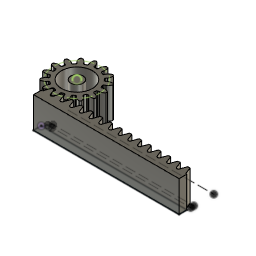
Rack and Gear (For creating a rack and gear) (Autodesk Fusion 360 design; units mm, degrees)
description: Spur Gear; Module: 2.0; Num Teeth: 15; Pressure Angle: 20.0; Backlash: 0.15 mm
Autodesk Fusion 360 part; units mm, degrees
sketch "Sketch1" plane through (0, 0, 0) normal (0, 0, 1) x (1, 0, 0)
  line L0 (0, 0) -> (94.2478, 0)
  line L1 (94.2478, 0) -> (94.2478, -5)
  line L2 (94.2478, -5) -> (0, -5)
  line L3 (0, -5) -> (0, 0)
  line L4 (0, 2.5) -> (94.2478, 2.5) construction
  line L5 (0, 4.5) -> (94.2478, 4.5) construction
  line L6 (0.7359, 0) -> (2.3737, 4.5)
  line L7 (2.3737, 4.5) -> (3.9094, 4.5)
  line L8 (3.9094, 4.5) -> (5.5473, 0)
  line L9 (0, 17.5) -> (94.2478, 17.5) construction
  point P0 (4.6374, 2.5)
  point P1 (1.6458, 2.5)
  point P2 (3.1416, 4.5)
  dimension "d7" = 94.2478
  dimension "d8" = 5
  dimension "d9" = 2.5
  dimension "d10" = 2
  dimension "d11" = 70
  dimension "d12" = 70
  dimension "d13" = 2.9916
  dimension "d14" = 3.1416
  dimension "d43" = 15
  constraint horizontal L0
  constraint vertical L1
  constraint horizontal L2
  constraint vertical L3
  constraint coincident L0.start L3.end
  constraint perpendicular L3 L4
  constraint horizontal L5
  constraint coincident L3 L4.start
  constraint coincident L3 L5.start
  constraint equal L0 L4
  constraint equal L0 L5
  constraint coincident L0 L6.start
  constraint coincident L5 L6.end
  constraint coincident L5 L7.end
  constraint coincident L0 L8.end
  constraint coincident L8 P0
  constraint coincident L4 P0
  constraint coincident L4 P1
  constraint coincident L6 P1
  constraint midpoint L7 P2
  constraint horizontal L9
  constraint equal L0 L9
  constraint coincident L3 L9.start
  measures "d7" distance of L0.start L0.end
  measures "d8" distance of L0.start L2.end
  measures "d9" distance of L0 L4
  measures "d10" distance of L4 L5
  measures "d11" angle of L0 L6
  measures "d12" angle of L0 L8
  measures "d13" distance of P0 P1
  measures "d14" distance of L3 P2
  measures "d43" distance of L4 L9
extrude "Extrude1" add sketch "Sketch1" along normal blind 20 contours L0 L1 L2 L3 makes body 1
extrude "Extrude2" add sketch "Sketch1" along normal blind 20 contours L0 L6 L7 L8 bodies 1
fillet "Fillet1" radius 0.76 2 edges at (0.7359, 0, 10) (5.5473, 0, 10) on bodies 1
pattern_linear "R-Pattern1" count 15 spacing 6.2832 along (1, 0, 0) of "Extrude2", "Fillet1"
copy_body "Body->Comp1" bodies 1 removing the originals makes body 2 in component "rack"
sketch "Sketch1 (2)" plane through (0, 0, 0) normal (0, 0, 1) x (1, 0, 0) in component "Shaft"
  circle A0 centre (0, 0) radius 4
  dimension "d34" = 8
  constraint coincident A0.centre origin
  measures "d34" diameter of A0
extrude "Extrude1'" add sketch "Sketch1 (2)" along normal blind 20 separate body makes body 3 in component "Shaft"
sketch "Sketch1 (3)" plane through (0, 0, 0) normal (0, 0, 1) x (1, 0, 0) in component "Spur Gear (15 teeth)"
  circle A0 centre (0, 0) radius 12.5492
  circle A1 centre (0, 0) radius 10
extrude "Extrude1''" add sketch "Sketch1 (3)" along normal blind 20 separate body makes body 4 in component "Spur Gear (15 teeth)"
sketch "Sketch2" plane through (0, 0, 0) normal (0, 0, 1) x (1, 0, 0) in component "Spur Gear (15 teeth)"
  spline S0 degree 5 poles (13.9988, -1.6471) (14.0073, -1.6481) (14.0244, -1.6499) (14.05, -1.6517) (14.0843, -1.6528) (14.1272, -1.6522) (14.1702, -1.6502) (14.2133, -1.6473) (14.2564, -1.644) (14.2995, -1.6403) (14.3427, -1.6363) (14.3859, -1.6318) (14.4291, -1.6268) (14.4723, -1.621) (14.5156, -1.6146) (14.5589, -1.6075) (14.6022, -1.5999) (14.6454, -1.5918) (14.6887, -1.5833) (14.732, -1.5744) (14.7753, -1.5652) (14.8186, -1.5555) (14.8619, -1.5454) (14.9052, -1.5349) (14.9484, -1.524) (14.9917, -1.5126) (15.0349, -1.5009) (15.0782, -1.4887) (15.1214, -1.4762) (15.1646, -1.4634) (15.2077, -1.4502) (15.2509, -1.4366) (15.294, -1.4227) (15.3372, -1.4084) (15.3803, -1.3938) (15.4233, -1.3789) (15.4664, -1.3636) (15.5094, -1.348) (15.5524, -1.332) (15.5953, -1.3157) (15.6383, -1.2991) (15.6811, -1.2822) (15.724, -1.265) (15.7668, -1.2475) (15.8096, -1.2296) (15.8524, -1.2115) (15.8951, -1.193) (15.9378, -1.1743) (15.9804, -1.1552) (16.023, -1.1359) (16.0655, -1.1162) (16.108, -1.0963) (16.1505, -1.0761) (16.1929, -1.0556) (16.2353, -1.0348) (16.2776, -1.0137) (16.3199, -0.9924) (16.3621, -0.9707) (16.4043, -0.9488) (16.4464, -0.9266) (16.4885, -0.9042) (16.5305, -0.8814) (16.5725, -0.8584) (16.6144, -0.8351) (16.6562, -0.8116) (16.698, -0.7878) (16.7398, -0.7637) (16.7814, -0.7394) (16.8231, -0.7148) (16.8646, -0.6899) (16.9061, -0.6648) (16.9393, -0.6445) (16.9641, -0.6292) (16.9806, -0.6189) (16.9889, -0.6138) knots 0 0 0 0 0 0 0.01428571 0.02857143 0.04285714 0.05714286 0.07142857 0.08571429 0.1 0.11428571 0.12857143 0.14285714 0.15714286 0.17142857 0.18571429 0.2 0.21428571 0.22857143 0.24285714 0.25714286 0.27142857 0.28571429 0.3 0.31428571 0.32857143 0.34285714 0.35714286 0.37142857 0.38571429 0.4 0.41428571 0.42857143 0.44285714 0.45714286 0.47142857 0.48571429 0.5 0.51428571 0.52857143 0.54285714 0.55714286 0.57142857 0.58571429 0.6 0.61428571 0.62857143 0.64285714 0.65714286 0.67142857 0.68571429 0.7 0.71428571 0.72857143 0.74285714 0.75714286 0.77142857 0.78571429 0.8 0.81428571 0.82857143 0.84285714 0.85714286 0.87142857 0.88571429 0.9 0.91428571 0.92857143 0.94285714 0.95714286 0.97142857 0.98571429 1 1 1 1 1 1
  spline S1 degree 5 poles (13.9988, 1.6471) (14.0073, 1.6481) (14.0244, 1.6499) (14.05, 1.6517) (14.0843, 1.6528) (14.1272, 1.6522) (14.1702, 1.6502) (14.2133, 1.6473) (14.2564, 1.644) (14.2995, 1.6403) (14.3427, 1.6363) (14.3859, 1.6318) (14.4291, 1.6268) (14.4723, 1.621) (14.5156, 1.6146) (14.5589, 1.6075) (14.6022, 1.5999) (14.6454, 1.5918) (14.6887, 1.5833) (14.732, 1.5744) (14.7753, 1.5652) (14.8186, 1.5555) (14.8619, 1.5454) (14.9052, 1.5349) (14.9484, 1.524) (14.9917, 1.5126) (15.0349, 1.5009) (15.0782, 1.4887) (15.1214, 1.4762) (15.1646, 1.4634) (15.2077, 1.4502) (15.2509, 1.4366) (15.294, 1.4227) (15.3372, 1.4084) (15.3803, 1.3938) (15.4233, 1.3789) (15.4664, 1.3636) (15.5094, 1.348) (15.5524, 1.332) (15.5953, 1.3157) (15.6383, 1.2991) (15.6811, 1.2822) (15.724, 1.265) (15.7668, 1.2475) (15.8096, 1.2296) (15.8524, 1.2115) (15.8951, 1.193) (15.9378, 1.1743) (15.9804, 1.1552) (16.023, 1.1359) (16.0655, 1.1162) (16.108, 1.0963) (16.1505, 1.0761) (16.1929, 1.0556) (16.2353, 1.0348) (16.2776, 1.0137) (16.3199, 0.9924) (16.3621, 0.9707) (16.4043, 0.9488) (16.4464, 0.9266) (16.4885, 0.9042) (16.5305, 0.8814) (16.5725, 0.8584) (16.6144, 0.8351) (16.6562, 0.8116) (16.698, 0.7878) (16.7398, 0.7637) (16.7814, 0.7394) (16.8231, 0.7148) (16.8646, 0.6899) (16.9061, 0.6648) (16.9393, 0.6445) (16.9641, 0.6292) (16.9806, 0.6189) (16.9889, 0.6138) knots 0 0 0 0 0 0 0.01428571 0.02857143 0.04285714 0.05714286 0.07142857 0.08571429 0.1 0.11428571 0.12857143 0.14285714 0.15714286 0.17142857 0.18571429 0.2 0.21428571 0.22857143 0.24285714 0.25714286 0.27142857 0.28571429 0.3 0.31428571 0.32857143 0.34285714 0.35714286 0.37142857 0.38571429 0.4 0.41428571 0.42857143 0.44285714 0.45714286 0.47142857 0.48571429 0.5 0.51428571 0.52857143 0.54285714 0.55714286 0.57142857 0.58571429 0.6 0.61428571 0.62857143 0.64285714 0.65714286 0.67142857 0.68571429 0.7 0.71428571 0.72857143 0.74285714 0.75714286 0.77142857 0.78571429 0.8 0.81428571 0.82857143 0.84285714 0.85714286 0.87142857 0.88571429 0.9 0.91428571 0.92857143 0.94285714 0.95714286 0.97142857 0.98571429 1 1 1 1 1 1
  arc A0 (16.9889, -0.6138) -> (16.9889, 0.6138) centre (0, 0) ccw
  line L0 (12.4533, -1.4665) -> (13.9988, -1.6471)
  line L1 (12.4533, 1.4665) -> (13.9988, 1.6471)
  line L2 (12.4533, -1.4665) -> (12.4533, 1.4665)
  point P0 (14.2076, -1.6476)
  point P1 (14.4187, -1.6279)
  point P2 (14.6312, -1.5944)
  point P3 (14.8446, -1.5494)
  point P4 (15.0588, -1.4941)
  point P5 (15.2735, -1.4293)
  point P6 (15.4885, -1.3555)
  point P7 (15.7036, -1.2732)
  point P8 (15.9188, -1.1826)
  point P9 (16.1337, -1.084)
  point P10 (16.3484, -0.9777)
  point P11 (16.5625, -0.8638)
  point P12 (16.7761, -0.7424)
  point P13 (14.2076, 1.6476)
  point P14 (14.4187, 1.6279)
  point P15 (14.6312, 1.5944)
  point P16 (14.8446, 1.5494)
  point P17 (15.0588, 1.4941)
  point P18 (15.2735, 1.4293)
  point P19 (15.4885, 1.3555)
  point P20 (15.7036, 1.2732)
  point P21 (15.9188, 1.1826)
  point P22 (16.1337, 1.084)
  point P23 (16.3484, 0.9777)
  point P24 (16.5625, 0.8638)
  point P25 (16.7761, 0.7424)
extrude "Extrude2'" add sketch "Sketch2" along normal blind 20 bodies 4 in component "Spur Gear (15 teeth)"
fillet "Fillet1'" radius 0.5 2 edges at (12.4631, -1.4676, 10) (12.4631, 1.4676, 10) on bodies 4 in component "Spur Gear (15 teeth)"
pattern_circular "C-Pattern1" count 15 over 360 about axis through (0, 0, 0) along (0, 0, 1) of "Extrude2'", "Fillet1'" in component "Spur Gear (15 teeth)"
sketch "Sketch3" plane through (0, 0, 0) normal (0, 0, 1) x (1, 0, 0) in component "Spur Gear (15 teeth)"
  circle A0 centre (0, 0) radius 15 construction
move_body "Move1" bodies 4 to x (0.999048, -0.043619, 0) y (0.043619, 0.999048, 0) z (0, 0, 1) at (0, 0, 0) in component "Spur Gear (15 teeth)"
component "Shaft" placed x (1, 0, 0) y (0, 1, 0) z (0, 0, 1) at (0.8804, 17.5, 0)
component "rack" placed x (1, 0, 0) y (0, 1, 0) z (0, 0, 1) at (0, 0, 0)
component "Spur Gear (15 teeth)" placed x (1, 0, 0) y (0, -1, 0) z (0, 0, -1) at (0.8804, 17.5, 20)
equation "module = 2 mm"
equation "pressureAngle = 20 deg"
equation "numberTeeth = 15"
equation "length = PI * module * numberTeeth"
equation "width = 20 mm"
equation "thickness = 5 mm"
equation "d7 = length"
equation "d8 = thickness"
equation "d9 = 1.25 * module"
equation "d10 = 1 * module"
equation "d11 = 90 deg - pressureAngle"
equation "d12 = 90 deg - pressureAngle"
equation "d13 = ( PI * module / 2 ) - backlash"
equation "d14 = PI * module / 2"
equation "d15 = width"
equation "d17 = width"
equation "d20 = 0.38 * module"
equation "d21 = numberTeeth"
equation "d23 = -PI * module"
equation "backlash = 0.15 mm"
equation "d35 = width"
equation "pitchDim = 30 mm"
equation "d43 = pitchDim / 2"
equation "distanceOne = 20.00 mm"
equation "taperAngle1 = 0.0 deg"
equation "Radius = 0.50 mm"
equation "countU = 15"
equation "d63 = 2 * 15 * PI mm"
